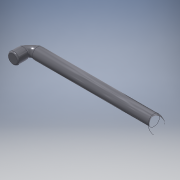
# Autodesk Inventor part: Solder Roll Support 3
Saved by Autodesk Inventor 2016 (Build 200138000, 138)
## iProperties
Created: 2017-09-04
Part Number: Solder Roll Support 3
Material: SAE 1020
Document SubType Name: Modeling
Designer: Zigunov
Stock Number: 0
Mass: 1729.01 g
Surface Area: 745.421 cm^2
Volume: 219.697 cm^3
Density: 7.87 g/cm^3
Appearance: Steel - Polished
Author: Zigunov
Autodesk Inventor part; units mm, degrees
ref_plane "YZ Plane" through (0, 0, 0) normal (1, 0, 0) x (0, 1, 0)
ref_plane "XZ Plane" through (0, 0, 0) normal (0, 1, 0) x (-1, 0, 0)
sketch "Sketch2" plane through (0, 0, 0) normal (0, 0, 1) x (1, 0, 0)
  line L0 (-26.25, -7) -> (26.25, -7) construction
  line L1 (26.25, -7) -> (26.25, -3)
  line L2 (23.25, 0) -> (-23.25, 0)
  line L3 (-26.25, -3) -> (-26.25, -7)
  arc A0 (-23.25, 0) -> (-26.25, -3) centre (-23.25, -3) ccw
  arc A1 (26.25, -3) -> (23.25, 0) centre (23.25, -3) ccw
  point P0 (0, 0)
  point P1 (26.25, 0)
  point P2 (-26.25, 0)
  point P3 (0, 0)
  dimension "d11" = 52.5
  dimension "d12" = 7
  dimension "d13" = 3
  constraints: 8 end point, 4 point on circle, 4 point on line, 4 tangent, 2 centre point, 2 parallel, 1 coincident, 1 equal radius, 1 horizontal, 1 midpoint, 1 perpendicular
  measures "d11" distance of point (26.25, 0) point (-26.25, 0)
  measures "d12" distance of point (-26.25, 0) L0.start
  measures "d13" radius of A0
ref_plane "Work Plane1" through (-26.25, -7, 0) normal (0, -1, 0) x (1, 0, 0)
sketch "Sketch3" plane through (-26.25, -7, 0) normal (0, -1, 0) x (1, 0, 0)
  circle A0 centre (0, 0) radius 2.25
  point P0 (26.25, 0)
  dimension "d14" = 4.5
  constraints: 1 centre point, 1 coincident
  measures "d14" diameter of A0
sweep "Sweep1" add profiles "Sketch3" path "Sketch2"
fillet "Fillet1" radius 0.5 6 edges at (28.5, -7, 0) (28.5, -3, 0) (23.25, 2.25, 0) (-23.25, 2.25, 0) (-28.5, -3, 0) (-28.5, -7, 0)
body "Solid2"
